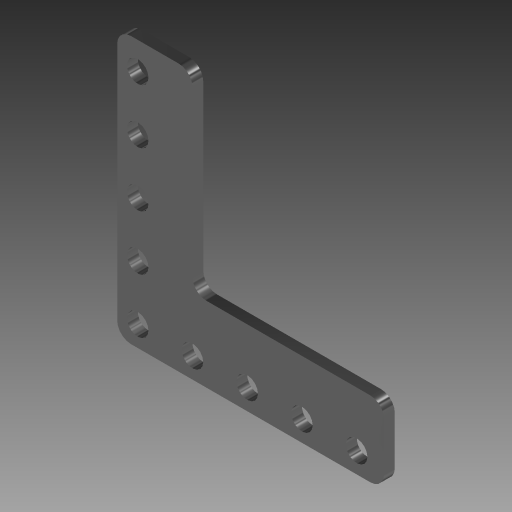
# Autodesk Inventor part: TTB Elevator L Gussets
Saved by Autodesk Inventor 2023 (Build 270158000, 158)
## iProperties
Created: 2022-12-30
Part Number: TTB Elevator L Gussets
Material: Generic
Document SubType Name: Modeling
Designer: Max Boord
Mass: 4.18378 g
Surface Area: 42.9761 cm^2
Volume: 4.18378 cm^3
Density: 1 g/cm^3
Appearance: Default
Mass: 8.91465 g
Surface Area: 35.9196 cm^2
Volume: 3.30172 cm^3
Density: 2.7 g/cm^3
Author: Max Boord
Mass: 6.92831 g
Surface Area: 65.1609 cm^2
Volume: 6.92831 cm^3
Mass: 8.83828 g
Surface Area: 82.9627 cm^2
Volume: 8.83828 cm^3
Mass: 4.17859 g
Surface Area: 42.9618 cm^2
Volume: 4.17859 cm^3
Autodesk Inventor part; units mm, degrees
ref_plane "YZ Plane" through (0, 0, 0) normal (1, 0, 0) x (0, 1, 0)
ref_plane "XZ Plane" through (0, 0, 0) normal (0, 1, 0) x (-1, 0, 0)
ref_plane "XY Plane" through (0, 0, 0) normal (0, 0, 1) x (1, 0, 0)
sketch "Sketch1" plane through (0, 0, 0) normal (0, 0, 1) x (1, 0, 0)
  line L0 (0, 0) -> (0, 69.85) construction
  line L1 (0, 69.85) -> (7.9375, 69.85) construction
  line L2 (7.9375, 69.85) -> (7.9375, 0) construction
  line L3 (7.9375, 69.85) -> (25.4, 69.85)
  line L4 (25.4, 69.85) -> (25.4, 17.4625)
  line L5 (25.4, 17.4625) -> (69.85, 17.4625)
  line L6 (69.85, 0) -> (0, 0) construction
  line L7 (25.4, 25.4) -> (69.85, 25.4)
  line L8 (69.85, 25.4) -> (69.85, 17.4625)
  circle A0 centre (12.7, 63.5) radius 2.4892
  circle A1 centre (12.7, 50.8) radius 2.4892
  circle A2 centre (12.7, 38.1) radius 2.4892
  circle A3 centre (12.7, 25.4) radius 2.4892
  circle A4 centre (12.7, 12.7) radius 2.4892
  circle A5 centre (25.4, 12.7) radius 2.4892
  circle A6 centre (38.1, 12.7) radius 2.4892
  circle A7 centre (50.8, 12.7) radius 2.4892
  circle A8 centre (63.5, 12.7) radius 2.4892
  line L9 (69.85, 7.9375) -> (7.9375, 7.9375)
  line L10 (69.85, 17.4625) -> (69.85, 7.9375)
  line L11 (69.85, 7.9375) -> (69.85, 0) construction
  line L12 (7.9375, 69.85) -> (7.9375, 7.9375)
  line L13 (12.7, 63.5) -> (12.7, 50.8) construction
  point P0 (16.6687, 69.85)
  dimension "d0" = 17.4625
  dimension "d3" = 25.4
  dimension "d4" = 4.9784
  dimension "d7" = 12.7
  dimension "d12" = 6.35
  dimension "d15" = 12.7
  dimension "d22" = 12.7
  dimension "d23" = 9.525
  dimension "d24" = 6.35
  dimension "d30" = 25.4
  dimension "d31" = 4.7625
  constraints: 28 end point, 9 centre point, 7 perpendicular, 4 vertical, 3 point on line, 2 collinear, 2 horizontal, 1 midpoint, 16 other
  measures "d0" distance between parallel lines of L4 L2
  measures "d3" distance between parallel lines of L6 L7
  measures "d4" diameter of A0
  measures "d7" distance of L13.start L13.end
  measures "d12" distance from line of L3 L13.start
  measures "d15" distance of A4.centre A5.centre
  measures "d22" distance from line of L6 A7.centre
  measures "d23" distance between parallel lines of L5 L9
  measures "d24" distance from line of A8.centre L10
  measures "d30" diameter of L0 L13
  measures "d31" distance from line of L13.start L2
extrude "Extrusion1" add sketch "Sketch1" along normal mid plane 2.5 contours L3 L4 L5 L10 L9 L12
extrude "Extrusion2" add sketch "Sketch1" along normal mid plane 2.5 contours L7 L8 L5 L4
fillet "Fillet1" radius 3.175 6 edges at (25.4, 69.85, 0) (7.9375, 69.85, 0) (7.9375, 7.9375, 0) (69.85, 7.9375, 0) (69.85, 25.4, 0) (25.4, 25.4, 0)
body "Solid1"
